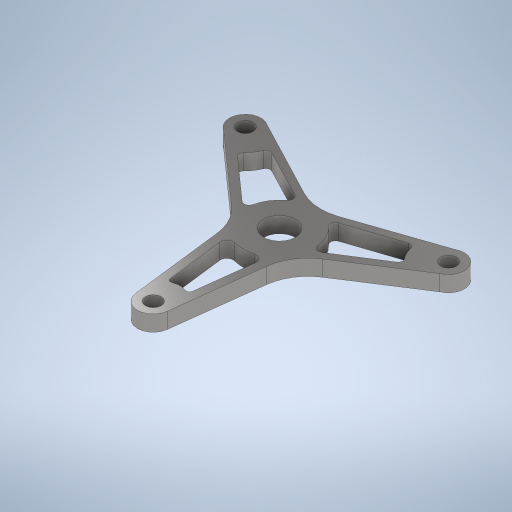
# Autodesk Inventor part: yoyo
Saved by Autodesk Inventor 2024 (Build 280153000, 153)
## iProperties
Created: 2024-02-02
Part Number: yoyo
Material: Stahl, galvanisiert
Document SubType Name: Modeling
Designer: ffogue
Density: 7.85 g/cm^3
Appearance: Galvanisiert
Author: ffogue
Autodesk Inventor part; units mm, degrees
ref_plane "YZ Plane" through (0, 0, 0) normal (1, 0, 0) x (0, 1, 0)
ref_plane "XZ Plane" through (0, 0, 0) normal (0, 1, 0) x (-1, 0, 0)
ref_plane "XY Plane" through (0, 0, 0) normal (0, 0, 1) x (1, 0, 0)
sketch "Skizze1" plane through (0, 0, 0) normal (0, 0, 1) x (1, 0, 0)
  line L0 (0, -80) -> (0, 80) construction
  line L1 (0, 0) -> (-126.7494, 85.2494) construction
  line L2 (0, 0) -> (174.2009, 85.2494) construction
  circle A0 centre (0, -80) radius 10
  line L3 (9.9263, -81.2121) -> (18.5, -11)
  line L4 (-9.9263, -81.2121) -> (-18.5, -11)
  arc A1 (11.1647, -27.3337) -> (6.298, -22.158) centre (7.3916, -26.0056) ccw
  arc A2 (-6.298, -22.158) -> (6.298, -22.158) centre (0, 0) ccw
  arc A3 (-6.298, -22.158) -> (-11.3621, -26.4905) centre (-7.3916, -26.0056) ccw
  circle A4 centre (0, 0) radius 10
  circle A5 centre (0, 0) radius 80 construction
  circle A6 centre (-66.3822, 44.6475) radius 10
  line L5 (-71.4336, 36.0171) -> (-18.5, -11)
  line L6 (-60.2936, 52.5803) -> (0, 21.0429)
  circle A7 centre (71.857, 35.1649) radius 10
  line L7 (18.5, -11) -> (75.6826, 25.9257)
  line L8 (0, 21.0429) -> (66.9086, 43.8548)
  line L9 (-11.3621, -26.4905) -> (-6.9853, -62.3337)
  arc A8 (-6.9853, -62.3337) -> (-4.1667, -63.9094) centre (-5, -62.0913) ccw
  arc A9 (4.1667, -63.9094) -> (-4.1667, -63.9094) centre (0, -73) ccw
  arc A10 (4.1667, -63.9094) -> (6.9853, -62.3337) centre (5, -62.0913) ccw
  line L10 (6.9853, -62.3337) -> (11.1647, -27.3337)
  dimension "d4" = 80
  dimension "d7" = 120
  dimension "d8" = 20
  dimension "d10" = 11
  dimension "d11" = 11
  dimension "d12" = 20
  dimension "d17" = 4
  dimension "d21" = 160
  dimension "d31" = 37
  dimension "d32" = 37
  dimension "d35" = 14
  dimension "d39" = 2
  dimension "d40" = 35.8432
  dimension "d41" = 7
  dimension "d43" = 35
  dimension "d71" = 10
  dimension "d77" = 10
  constraints: 24 point on circle, 22 end point, 11 centre point, 7 tangent, 4 coincident, 3 equal radius, 3 point on line, 2 horizontal alignment, 2 midpoint, 2 symmetric about line, 1 concentric, 1 equal length, 1 parallel, 1 vertical, 1 vertical alignment
  measures "d4" distance of L0.start L1.start
  measures "d7" angle of L2 L1
  measures "d8" diameter of A0
  measures "d10" vertical distance of L3.end L1.start
  measures "d11" vertical distance of L1.start L4.end
  measures "d12" diameter of A4
  measures "d17" radius of A3
  measures "d21" diameter of A5
  measures "d31" distance of L3.end L4.end
  measures "d32" distance of L6.end L4.end
  measures "d35" angle of L6 L5
  measures "d39" radius of A8
  measures "d40" vertical distance of L9.start L9.end
  measures "d41" distance of L0.start A9.centre
  measures "d43" vertical distance of L10.start L10.end
  measures "d71" distance of A8.centre A10.centre
  measures "d77" radius of A9
extrude "Extrusion2" add sketch "Skizze1" along normal blind 10 contours A0 | A0 L4 L5 A6 L6 L8 A7 L7 L3 | A6 | A7 | L10 A10 A9 A8 L9 A3 A2 A1
sketch "Skizze4" plane through (0, 0, 10) normal (0, 0, 1) x (1, 0, 0)
  arc A0 (-9.9263, -81.2121) -> (9.9263, -81.2121) centre (0, -80) ccw projected
  point P0 (0, 0)
  constraints: 1 coincident
hole "Bohrung1" at (0, -80, 10) direction (0, 0, -1) diameter 10 depth 10
sketch "Skizze5" plane through (0, 0, 10) normal (0, 0, 1) x (1, 0, 0)
  arc A0 (-60.2936, 52.5803) -> (-71.4336, 36.0171) centre (-66.3822, 44.6475) ccw projected
  arc A1 (75.6826, 25.9257) -> (66.9086, 43.8548) centre (71.857, 35.1649) ccw projected
  point P0 (0, 0)
  constraints: 2 coincident
hole "Bohrung2" at (-66.3822, 44.6475, 10) at (71.857, 35.1649, 10) direction (0, 0, -1) diameter 10 depth 10
fillet "Rundung1" radius 30 3 edges at (0, 21.0429, 5) (18.5, -11, 5) (-18.5, -11, 5)
sketch "Skizze6" plane through (0, 0, 10) normal (0, 0, 1) x (1, 0, 0)
  circle A0 centre (-66.3822, 44.6475) radius 5 projected
  line L0 (0, 0) -> (-66.3822, 44.6475) construction
  arc A1 (-12.9165, 17.7381) -> (-21.4837, 4.4641) centre (0, 0) ccw
  circle A2 centre (0, 0) radius 10 projected
  arc A3 (-12.9165, 17.7381) -> (-13.2992, 22.9189) centre (-14.7162, 20.2097) ccw
  line L1 (-13.2992, 22.9189) -> (-43.9218, 38.9365)
  arc A4 (-43.9218, 38.9365) -> (-47.8486, 37.4608) centre (-45.2257, 36.4437) ccw
  arc A5 (-52.7377, 30.1917) -> (-47.8486, 37.4608) centre (-66.3822, 44.6475) ccw
  arc A6 (-52.7377, 30.1917) -> (-52.6749, 26.0427) centre (-50.8067, 28.1459) ccw
  line L2 (-52.6749, 26.0427) -> (-26.5076, 2.8001)
  arc A7 (-26.5076, 2.8001) -> (-21.4837, 4.4641) centre (-24.4772, 5.0861) ccw
  line L3 (-71.4336, 36.0171) -> (-26.9812, -3.4668) projected
  line L4 (-11.4042, 27.008) -> (-60.2936, 52.5803) projected
  dimension "d61" = 10
  dimension "d62" = 5
  dimension "d63" = 5
  dimension "d64" = 18
  dimension "d66" = 25
  dimension "d67" = 35
  dimension "d68" = 5
  constraints: 12 point on circle, 7 tangent, 6 centre point, 6 end point, 2 concentric, 2 equal radius, 2 parallel
  measures "d61" distance of A6.centre A4.centre
  measures "d62" distance from line of L0 A4.centre
  measures "d63" distance from line of A6.centre L0
  measures "d64" distance of A7.centre A3.centre
  measures "d66" distance of L0.start A7.centre
  measures "d67" distance of A7.centre A6.centre
  measures "d68" distance between parallel lines of L3 L2
extrude "Extrusion4" cut sketch "Skizze6" against normal blind 10 contours A1 A7 L2 A6 A5 A4 L1 A3
pattern_circular "Runde Anordnung1" count 2 over 120 about axis through (0, 0, 0) along (0, 0, -1) of "Extrusion4"
extrude "Extrusion5" cut sketch "Skizze1" along normal blind 10 contours L10 A10 A9 A8 L9 A3 A2 A1
equation "\"d32\" = d31"
equation "\"d62\" = 0.5 * d61"
equation "\"d63\" = 0.5 * d61"
